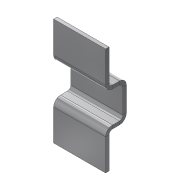
# Autodesk Inventor part: M18 - Aluminum Bracket
Saved by Autodesk Inventor 2016 (Build 200138000, 138)
## iProperties
Created: 2017-02-27
Part Number: M18 - Aluminum Bracket
Material: Aluminum 6061
Document SubType Name: Sheet Metal
Designer: Fernando
Mass: 1.5562 g
Surface Area: 12.5959 cm^2
Volume: 0.576372 cm^3
Density: 2.7 g/cm^3
Sheet Metal Rule: Default
Sheet Metal Width: 2869,500 mm
Sheet Metal Length: 526520,233 mm^2
Appearance: Aluminum - Dark
SurfaceArea_m2: 0
Author: Fernando
Autodesk Inventor part; units mm, degrees
note: some values were not read from the file. Chosen so that the rebuilt part matches the saved one: flange form of "Plate2".
ref_plane "YZ Plane" through (0, 0, 0) normal (1, 0, 0) x (0, 1, 0)
ref_plane "XZ Plane" through (0, 0, 0) normal (0, 1, 0) x (-1, 0, 0)
ref_plane "XY Plane" through (0, 0, 0) normal (0, 0, 1) x (1, 0, 0)
sketch "Sketch8" plane through (0, 0, 0) normal (1, 0, 0) x (0, 1, 0)
  line L0 (0, 15.5) -> (0, 5.5)
  line L1 (0, 5.5) -> (5, 5.5)
  line L2 (5, 5.5) -> (5, -5.5)
  line L3 (5, -5.5) -> (0, -5.5)
  line L4 (0, -5.5) -> (0, -15.5)
  point P0 (0, 0)
  point P1 (5, 0)
  dimension "d39" = 11
  dimension "d40" = 5
  dimension "d41" = 10
  dimension "d42" = 10
  measures "d39" distance of L1.end L2.end
  measures "d40" distance of L0.end L1.end
  measures "d41" distance of L0.start L0.end
  measures "d42" distance of L3.end L4.end
contour flange "Contour Flange1" sketch "Sketch8" thickness 1 bend radius 1 width 15 along (1, 0, 0) mid plane no both sides no wall seen from (0, 0, 10.5) lies toward (0, -1, 0) curves L0 L1 L2 L3 L4
bend "Bend1"
corner "Corner1"
equation "\"d29\" = BendReliefWidth"
equation "\"d30\" = BendReliefDepth"
equation "\"d31\" = MinimumRemnant"
equation "\"d32\" = BendRadius"
equation "\"d34\" = BendRadius"
equation "\"d36\" = CornerReliefSize"
equation "\"d37\" = GapSize"
equation "\"d38\" = JacobiRadiusSize"
equation "\"BendRadius\" = Thickness"
equation "\"BendReliefWidth\" = Thickness"
equation "\"BendReliefDepth\" = 0.5 * Thickness"
equation "\"CornerReliefSize\" = 4 * Thickness"
equation "\"MinimumRemnant\" = 2 * Thickness"
equation "\"TransitionRadius\" = BendRadius"
equation "\"JacobiRadiusSize\" = Thickness"
equation "\"GapSize\" = Thickness"
equation "\"d23\" = BendRadius"
equation "\"Thickness\" = 1"
body "Solid3"
